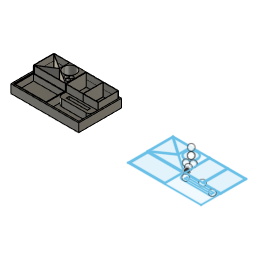
Desk Organizer v13 (Autodesk Fusion 360 design; units mm, degrees)
Autodesk Fusion 360 part; units mm, degrees
sketch "Sketch1" plane through (0, 0, 0) normal (0, 0, 1) x (1, 0, 0)
  line L0 (125, -80) -> (-125, -80)
  line L1 (-125, -80) -> (-125, 80)
  line L2 (-125, 80) -> (125, 80)
  line L3 (125, 80) -> (125, -80)
  line L4 (125, -80) -> (-125, 80) construction
  line L5 (-125, -80) -> (125, 80) construction
  dimension "d1" = 250
  constraint horizontal L0
  constraint perpendicular L0 L1
  constraint parallel L0 L2
  constraint parallel L1 L3
  constraint coincident L4 origin
  constraint coincident L5 origin
  measures "d1" distance of L1.end L2.end
extrude "Extrude1" add sketch "Sketch1" along normal blind 30 makes body 1
sketch "Sketch2" plane through (0, 0, 30) normal (0, 0, 1) x (-1, 0, 0)
  line L0 (-125, -80) -> (125, -80)
  line L1 (125, -80) -> (125, 80)
  line L2 (125, 80) -> (-125, 80)
  line L3 (-125, 80) -> (-125, -80)
  line L4 (119.192, -76.1203) -> (-119.192, -76.1203)
  line L5 (-119.192, -76.1203) -> (-119.192, 76.1203)
  line L6 (-119.192, 76.1203) -> (119.192, 76.1203)
  line L7 (119.192, 76.1203) -> (119.192, -76.1203)
  line L8 (119.192, -76.1203) -> (-119.192, 76.1203) construction
  line L9 (-119.192, -76.1203) -> (119.192, 76.1203) construction
  constraint horizontal L4
  constraint perpendicular L4 L5
  constraint parallel L4 L6
  constraint parallel L5 L7
  constraint coincident L8 origin
  constraint coincident L9 origin
extrude "Extrude2" cut sketch "Sketch2" against normal blind 26 contours L4 L5 L6 L7 bodies 1
sketch "Sketch3" plane through (0, 0, 4) normal (0, 0, 1) x (-1, 0, 0)
  line L0 (119.192, 76.1203) -> (-119.192, 76.1203)
  line L1 (-119.192, 76.1203) -> (-119.192, -76.1203)
  line L2 (-119.192, -76.1203) -> (119.192, -76.1203)
  line L3 (119.192, -76.1203) -> (119.192, 76.1203)
  line L4 (2.1554, -1.5872) -> (116.2965, -1.5872)
  line L5 (116.2965, -1.5872) -> (116.2965, -74.3239)
  line L6 (116.2965, -74.3239) -> (2.1554, -74.3239)
  line L7 (2.1554, -74.3239) -> (2.1554, -1.5872)
  line L8 (2.1554, -1.5872) -> (116.2965, -74.3239) construction
  line L9 (116.2965, -1.5872) -> (2.1554, -74.3239) construction
  point P0 (59.2259, -37.9555)
  constraint horizontal L4
  constraint perpendicular L4 L5
  constraint parallel L4 L6
  constraint parallel L5 L7
  constraint coincident L8 P0
  constraint coincident L9 P0
extrude "Extrude3" add sketch "Sketch3" along normal blind 50 separate body contours L4 L5 L6 L7 makes body 2
sketch "Sketch4" plane through (0, 0, 30) normal (0, 0, 1) x (-1, 0, 0)
  line L0 (-119.192, -76.1203) -> (-119.192, 76.1203)
  line L1 (-119.192, 76.1203) -> (119.192, 76.1203)
  line L2 (119.192, 76.1203) -> (119.192, -76.1203)
  line L3 (119.192, -76.1203) -> (-119.192, -76.1203)
  line L4 (-125, -80) -> (125, -80)
  line L5 (125, -80) -> (125, 80)
  line L6 (125, 80) -> (-125, 80)
  line L7 (-125, 80) -> (-125, -80)
sketch "Sketch5" plane through (0, 0, 54) normal (0, 0, 1) x (-1, 0, 0)
  line L0 (2.1554, -74.3239) -> (116.2965, -74.3239)
  line L1 (116.2965, -74.3239) -> (116.2965, -1.5872)
  line L2 (116.2965, -1.5872) -> (2.1554, -1.5872)
  line L3 (2.1554, -1.5872) -> (2.1554, -74.3239)
  line L4 (115, -72.3079) -> (115, -2.8697)
  line L5 (115, -2.8697) -> (5, -2.8697)
  line L6 (5, -2.8697) -> (5, -72.3079)
  line L7 (5, -72.3079) -> (115, -72.3079)
  line L8 (115, -72.3079) -> (5, -2.8697)
  line L9 (5, -72.3079) -> (115, -2.8697)
  constraint parallel L1 L4
  constraint perpendicular L4 L5
  constraint perpendicular L5 L6
  constraint perpendicular L4 L7
extrude "Extrude4" cut sketch "Sketch5" against normal blind 45 contours L4 L8 L9 bodies 2
sketch "Sketch6" plane through (0, 0, 54) normal (0, 0, 1) x (-1, 0, 0)
  line L0 (60, -37.5888) -> (115, -2.8697)
  line L1 (115, -2.8697) -> (115, -72.3079)
  line L2 (115, -72.3079) -> (60, -37.5888)
  line L3 (2.1554, -74.3239) -> (116.2965, -74.3239)
  line L4 (116.2965, -74.3239) -> (116.2965, -1.5872)
  line L5 (116.2965, -1.5872) -> (2.1554, -1.5872)
  line L6 (2.1554, -1.5872) -> (2.1554, -74.3239)
  line L7 (59.2259, -37.1001) -> (3.961, -2.9832)
  line L8 (3.961, -2.9832) -> (113.0235, -2.8515)
  line L9 (113.0235, -2.8515) -> (59.2259, -37.1001)
extrude "Extrude5" cut sketch "Sketch6" against normal blind 45 contours L7 L8 L9 bodies 2
sketch "Sketch7" plane through (0, 0, 54) normal (0, 0, 1) x (-1, 0, 0)
  line L0 (59.2259, -37.1001) -> (3.961, -2.9832)
  line L1 (3.961, -2.9832) -> (113.0235, -2.8515)
  line L2 (113.0235, -2.8515) -> (59.2259, -37.1001)
  line L3 (60, -37.5888) -> (115, -2.8697)
  line L4 (115, -2.8697) -> (115, -72.3079)
  line L5 (115, -72.3079) -> (60, -37.5888)
  line L6 (2.1554, -74.3239) -> (116.2965, -74.3239)
  line L7 (116.2965, -74.3239) -> (116.2965, -1.5872)
  line L8 (116.2965, -1.5872) -> (2.1554, -1.5872)
  line L9 (2.1554, -1.5872) -> (2.1554, -74.3239)
  line L10 (60, -38.3558) -> (60, -73.2667)
  line L11 (60, -73.2667) -> (115, -73.2667)
  line L12 (115, -73.2667) -> (60, -38.3558)
  constraint vertical L10
  constraint perpendicular L10 L11
extrude "Extrude6" cut sketch "Sketch7" against normal blind 45 contours L10 L11 L12 bodies 2
sketch "Sketch8" plane through (0, 0, 54) normal (0, 0, 1) x (-1, 0, 0)
  line L0 (60, -73.2667) -> (60, -38.3558)
  line L1 (60, -38.3558) -> (115, -73.2667)
  line L2 (115, -73.2667) -> (60, -73.2667)
  line L3 (59.2259, -37.1001) -> (3.961, -2.9832)
  line L4 (3.961, -2.9832) -> (113.0235, -2.8515)
  line L5 (113.0235, -2.8515) -> (59.2259, -37.1001)
  line L6 (60, -37.5888) -> (115, -2.8697)
  line L7 (115, -2.8697) -> (115, -72.3079)
  line L8 (115, -72.3079) -> (60, -37.5888)
  line L9 (2.1554, -74.3239) -> (116.2965, -74.3239)
  line L10 (116.2965, -74.3239) -> (116.2965, -1.5872)
  line L11 (116.2965, -1.5872) -> (2.1554, -1.5872)
  line L12 (2.1554, -1.5872) -> (2.1554, -74.3239)
  circle A0 centre (35.6462, -50.553) radius 22.3607
extrude "Extrude7" cut sketch "Sketch8" against normal blind 45 contours A0 bodies 2
move_body "Move1" bodies 2 to x (1, 0, 0) y (0, 1, 0) z (0, 0, 1) at (283.173, -5.0322, 0)
sketch "Sketch9" plane through (0, 0, 54) normal (0, 0, 1) x (-1, 0, 0)
  circle A0 centre (-247.5268, -45.5208) radius 22.3607
  line L0 (-223.173, -68.2344) -> (-223.173, -33.3236)
  line L1 (-223.173, -33.3236) -> (-168.173, -68.2344)
  line L2 (-168.173, -68.2344) -> (-223.173, -68.2344)
  line L3 (-223.947, -32.0679) -> (-279.212, 2.049)
  line L4 (-279.212, 2.049) -> (-170.1495, 2.1807)
  line L5 (-170.1495, 2.1807) -> (-223.947, -32.0679)
  line L6 (-223.173, -32.5565) -> (-168.173, 2.1626)
  line L7 (-168.173, 2.1626) -> (-168.173, -67.2756)
  line L8 (-168.173, -67.2756) -> (-223.173, -32.5565)
  line L9 (-281.0176, -69.2917) -> (-166.8765, -69.2917)
  line L10 (-166.8765, -69.2917) -> (-166.8765, 3.4451)
  line L11 (-166.8765, 3.4451) -> (-281.0176, 3.4451)
  line L12 (-281.0176, 3.4451) -> (-281.0176, -69.2917)
  circle A1 centre (-261.4315, -18.5457) radius 6.2199
  circle A2 centre (-272.1085, -27.4432) radius 6.2744
  circle A3 centre (-273.71, -12.3175) radius 6.3191
extrude "Extrude8" cut sketch "Sketch9" against normal blind 45 contours A1 | A2 | A3 bodies 2
move_body "Move2" bodies 2 to x (1, 0, 0) y (0, 1, 0) z (0, 0, 1) at (-284.7373, 5.4237, 0)
sketch "Sketch10" plane through (0, 0, 54) normal (0, 0, 1) x (-1, 0, 0)
  circle A0 centre (12.6289, -32.8669) radius 6.2744
  circle A1 centre (23.3058, -23.9694) radius 6.2199
  circle A2 centre (11.0273, -17.7412) radius 6.3191
  circle A3 centre (37.2105, -50.9445) radius 22.3607
  line L0 (61.5643, -73.6581) -> (61.5643, -38.7472)
  line L1 (61.5643, -38.7472) -> (116.5643, -73.6581)
  line L2 (116.5643, -73.6581) -> (61.5643, -73.6581)
  line L3 (60.7903, -37.4916) -> (5.5253, -3.3747)
  line L4 (5.5253, -3.3747) -> (114.5878, -3.2429)
  line L5 (114.5878, -3.2429) -> (60.7903, -37.4916)
  line L6 (61.5643, -37.9802) -> (116.5643, -3.2611)
  line L7 (116.5643, -3.2611) -> (116.5643, -72.6993)
  line L8 (116.5643, -72.6993) -> (61.5643, -37.9802)
  line L9 (3.7197, -74.7154) -> (117.8608, -74.7154)
  line L10 (117.8608, -74.7154) -> (117.8608, -1.9786)
  line L11 (117.8608, -1.9786) -> (3.7197, -1.9786)
  line L12 (3.7197, -1.9786) -> (3.7197, -74.7154)
  line L13 (-116.6264, -1.9786) -> (-1.9597, -1.9786)
  line L14 (-1.9597, -1.9786) -> (-1.9597, -74.7154)
  line L15 (-1.9597, -74.7154) -> (-116.6264, -74.7154)
  line L16 (-116.6264, -74.7154) -> (-116.6264, -1.9786)
  line L17 (-116.6264, -1.9786) -> (-1.9597, -74.7154) construction
  line L18 (-1.9597, -1.9786) -> (-116.6264, -74.7154) construction
  point P0 (-59.2931, -38.347)
  constraint horizontal L13
  constraint perpendicular L13 L14
  constraint parallel L13 L15
  constraint parallel L14 L16
  constraint coincident L17 P0
  constraint coincident L18 P0
  constraint midpoint L17 P0
extrude "Extrude9" add sketch "Sketch10" against normal blind 49 separate body contours L13 L14 L15 L16 makes body 3
sketch "Sketch11" plane through (0, 0, 54) normal (0, 0, 1) x (-1, 0, 0)
  line L0 (-116.6264, -74.7154) -> (-1.9597, -74.7154)
  line L1 (-1.9597, -74.7154) -> (-1.9597, -1.9786)
  line L2 (-1.9597, -1.9786) -> (-116.6264, -1.9786)
  line L3 (-116.6264, -1.9786) -> (-116.6264, -74.7154)
  line L4 (-3.5608, -73.4896) -> (-62.607, -73.4896)
  line L5 (-62.607, -73.4896) -> (-62.607, -3.1642)
  line L6 (-62.607, -3.1642) -> (-3.5608, -3.1642)
  line L7 (-3.5608, -3.1642) -> (-3.5608, -73.4896)
  constraint horizontal L4
  constraint vertical L5
  constraint horizontal L6
  constraint vertical L7
extrude "Extrude10" cut sketch "Sketch11" against normal blind 45 contours L4 L5 L6 L7 bodies 3
sketch "Sketch12" plane through (0, 0, 54) normal (0, 0, 1) x (-1, 0, 0)
  line L0 (-62.607, -73.4896) -> (-62.607, -3.1642)
  line L1 (-62.607, -3.1642) -> (-3.5608, -3.1642)
  line L2 (-3.5608, -3.1642) -> (-3.5608, -73.4896)
  line L3 (-3.5608, -73.4896) -> (-62.607, -73.4896)
  line L4 (-116.6264, -74.7154) -> (-1.9597, -74.7154)
  line L5 (-1.9597, -74.7154) -> (-1.9597, -1.9786)
  line L6 (-1.9597, -1.9786) -> (-116.6264, -1.9786)
  line L7 (-116.6264, -1.9786) -> (-116.6264, -74.7154)
  line L8 (-63.6611, -73.4896) -> (-116, -73.4896)
  line L9 (-116, -73.4896) -> (-116, -3.3521)
  line L10 (-116, -3.3521) -> (-63.6611, -3.3521)
  line L11 (-63.6611, -3.3521) -> (-63.6611, -73.4896)
  constraint horizontal L8
  constraint vertical L9
  constraint horizontal L10
  constraint vertical L11
extrude "Extrude11" cut sketch "Sketch12" against normal blind 45 contours L8 L9 L10 L11 bodies 3
sketch "Sketch13" plane through (0, 0, 30) normal (0, 0, 1) x (-1, 0, 0)
  line L0 (-3.0546, 2.517) -> (-115, 2.517)
  line L1 (-115, 2.517) -> (-115, 17.5)
  line L2 (-102.5, 30) -> (-15.5546, 30)
  line L3 (-3.0546, 17.5) -> (-3.0546, 2.517)
  arc A0 (-3.0546, 17.5) -> (-15.5546, 30) centre (-15.5546, 17.5) ccw
  arc A1 (-102.5, 30) -> (-115, 17.5) centre (-102.5, 17.5) ccw
  dimension "d24" = 12.5
  constraint horizontal L0
  constraint vertical L1
  constraint horizontal L2
  constraint vertical L3
  constraint tangent L2 A0
  constraint tangent L3 A0
  constraint tangent L1 A1
  constraint tangent L2 A1
  constraint equal A0 A1
  measures "d24" radius of A0
extrude "Extrude12" add sketch "Sketch13" against normal blind 25 separate body makes body 4
sketch "Sketch14" plane through (0, 0, 30) normal (0, 0, 1) x (-1, 0, 0)
  line L0 (-22.0307, 10) -> (-97.0307, 10)
  line L1 (-97.0307, 10) -> (-97.0307, 20)
  line L2 (-97.0307, 20) -> (-22.0307, 20)
  line L3 (-22.0307, 20) -> (-22.0307, 10)
  constraint horizontal L0
  constraint vertical L1
  constraint horizontal L2
  constraint vertical L3
extrude "Extrude13" cut sketch "Sketch14" against normal blind 20 bodies 4
sketch "Sketch15" plane through (0, 0, 30) normal (0, 0, 1) x (-1, 0, 0)
  line L0 (116.1282, 2.9693) -> (1.7275, 2.9693)
  line L1 (1.7275, 2.9693) -> (1.7275, 73.433)
  line L2 (1.7275, 73.433) -> (116.1282, 73.433)
  line L3 (116.1282, 73.433) -> (116.1282, 2.9693)
  constraint horizontal L0
  constraint vertical L1
  constraint horizontal L2
  constraint vertical L3
sketch "Sketch16" plane through (0, 0, 30) normal (0, 0, 1) x (-1, 0, 0)
  line L0 (113.46, 5.4) -> (5.0422, 5.4)
  line L1 (5.0422, 5.4) -> (5.0422, 70.1017)
  line L2 (5.0422, 70.1017) -> (113.46, 70.1017)
  line L3 (113.46, 70.1017) -> (113.46, 5.4)
  constraint horizontal L0
  constraint vertical L1
  constraint horizontal L2
  constraint vertical L3
move_body "Move3" bodies 1 to x (1, 0, 0) y (0, 1, 0) z (0, 0, 1) at (-266.4429, 0, 1.5616)
move_body "Move4" bodies 2 to x (1, 0, 0) y (0, 1, 0) z (0, 0, 1) at (-55.2047, 106.1335, 0)
move_body "Move5" bodies 3 to x (1, 0, 0) y (0, 1, 0) z (0, 0, 1) at (-11.6109, 104.6452, 0)
move_body "Move6" bodies 4 to x (1, 0, 0) y (0, 1, 0) z (0, 0, 1) at (5.9394, -97.6743, 0)
move_body "Move8" bodies 3 to x (1, 0, 0) y (0, 1, 0) z (0, 0, 1) at (-255.7495, -105.647, 0)
move_body "Move9" bodies 2 to x (1, 0, 0) y (0, 1, 0) z (0, 0, 1) at (-209.1872, -107.0558, 0)
move_body "Move11" bodies 4 to x (1, 0, 0) y (0, 1, 0) z (0, 0, 1) at (-273.4479, 96.4393, 0)
move_body "Move12" bodies 2 to x (1, 0, 0) y (0, 1, 0) z (0, 0, 1) at (-2.937, 1.7568, 0)
move_body "Move13" bodies 3 to x (1, 0, 0) y (0, 1, 0) z (0, 0, 1) at (-4.7566, 1.6446, 0)
move_body "Move15" bodies 4 to x (1, 0, 0) y (0, 1, 0) z (0, 0, 1) at (-4.1785, 5.2913, 0)
move_face "OffsetFaces1" offset 7 1 faces at (-147.2509, 25.3734, 22.8949) on bodies 1
move_face "OffsetFaces2" offset -8 1 faces at (-141.4429, 26.6667, 11.5616) on bodies 1
move_face "OffsetFaces3" offset -1 1 faces at (-391.4429, -26.6667, 11.5616) on bodies 1
move_face "OffsetFaces4" offset 9 1 faces at (-231.3789, -76.1203, 22.8949) on bodies 1
move_face "OffsetFaces5" offset -8 1 faces at (-229.7762, -80, 21.5616) on bodies 1
sketch "Sketch17" plane through (0, 0, 5.5616) normal (0, 0, 1) x (-1, 0, 0)
  line L0 (385.6348, 67.1203) -> (154.2509, 67.1203)
  line L1 (154.2509, 67.1203) -> (154.2509, -76.1203)
  line L2 (154.2509, -76.1203) -> (385.6348, -76.1203)
  line L3 (385.6348, -76.1203) -> (385.6348, 67.1203)
  line L4 (385, -2) -> (271, -2)
  line L5 (271, -2) -> (271, 66.2697)
  line L6 (271, 66.2697) -> (385, 66.2697)
  line L7 (385, 66.2697) -> (385, -2)
  constraint horizontal L4
  constraint vertical L5
  constraint horizontal L6
  constraint vertical L7
extrude "Extrude16" add sketch "Sketch17" along normal blind 25 separate body contours L4 L5 L6 L7 makes body 5
move_body "Move17" bodies 5 to x (1, 0, 0) y (0, 1, 0) z (0, 0, 1) at (-11.9716, -62.1549, -50.1833)
move_body "Move18" bodies 5 to x (1, 0, 0) y (0, 1, 0) z (0, 0, 1) at (-119.3378, 20.5362, 0)
sketch "Sketch18" plane through (0, 0, -19.6217) normal (0, 0, 1) x (-1, 0, 0)
  line L0 (516.3095, 107.8885) -> (402.3095, 107.8885)
  line L1 (402.3095, 107.8885) -> (402.3095, 39.6188)
  line L2 (402.3095, 39.6188) -> (516.3095, 39.6188)
  line L3 (516.3095, 39.6188) -> (516.3095, 107.8885)
  line L4 (513.6378, 41.8099) -> (405, 41.8099)
  line L5 (405, 41.8099) -> (405, 106.0721)
  line L6 (405, 106.0721) -> (513.6378, 106.0721)
  line L7 (513.6378, 106.0721) -> (513.6378, 41.8099)
  constraint horizontal L4
  constraint vertical L5
  constraint horizontal L6
  constraint vertical L7
extrude "Extrude17" cut sketch "Sketch18" against normal blind 22 contours L4 L5 L6 L7 bodies 5
move_body "Move19" bodies 5 to x (1, 0, 0) y (0, 1, 0) z (0, 0, 1) at (131.831, 41.6514, 50)
sketch "Sketch19" plane through (0, 0, 0) normal (0, 0, 1) x (1, 0, 0)
  line L0 (288.7232, -75.5137) -> (28.7232, -75.5137)
  line L1 (28.7232, -75.5137) -> (28.7232, 84.4863)
  line L2 (28.7232, 84.4863) -> (288.7232, 84.4863)
  line L3 (288.7232, 84.4863) -> (288.7232, -75.5137)
  line L4 (158.7232, 84.4863) -> (288.7232, 84.4863)
  line L5 (288.7232, 84.4863) -> (288.7232, -5.5137)
  line L6 (288.7232, -5.5137) -> (158.7232, -5.5137)
  line L7 (158.7232, -5.5137) -> (158.7232, 84.4863)
  line L8 (28.7232, 84.4863) -> (158.7232, 84.4863)
  line L9 (158.7232, 84.4863) -> (158.7232, -5.5137)
  line L10 (158.7232, -5.5137) -> (28.7232, -5.5137)
  line L11 (28.7232, -5.5137) -> (28.7232, 84.4863)
  line L12 (28.7232, 84.4863) -> (158.7232, -5.5137)
  line L13 (28.7232, -5.5137) -> (93.7232, 39.4863)
  line L14 (93.7232, 39.4863) -> (93.7232, 84.4863)
  circle A0 centre (119.0143, 58.7272) radius 22.3607
  circle A1 centre (132.504, 27.4364) radius 9.2562
  circle A2 centre (148.2489, 37.2769) radius 8.7724
  circle A3 centre (150.0202, 17.9895) radius 8.6173
  line L15 (223.7232, 84.4863) -> (223.7232, -5.5137)
  line L16 (31.661, -7.9668) -> (157.827, -7.9668)
  line L17 (157.827, -7.9668) -> (157.827, -73.0925)
  line L18 (157.827, -73.0925) -> (31.661, -73.0925)
  line L19 (31.661, -73.0925) -> (31.661, -7.9668)
  line L20 (164.4427, -7.9668) -> (283.7232, -7.9668)
  line L21 (283.7232, -7.9668) -> (283.7232, -18.0137)
  line L22 (271.2232, -30.5137) -> (176.9427, -30.5137)
  line L23 (164.4427, -18.0137) -> (164.4427, -7.9668)
  arc A4 (164.4427, -18.0137) -> (176.9427, -30.5137) centre (176.9427, -18.0137) ccw
  arc A5 (271.2232, -30.5137) -> (283.7232, -18.0137) centre (271.2232, -18.0137) ccw
  point P0 (158.7232, 4.4863)
  dimension "d43" = 12.5
  constraint horizontal L0
  constraint perpendicular L0 L1
  constraint parallel L0 L2
  constraint parallel L1 L3
  constraint horizontal L4
  constraint vertical L5
  constraint horizontal L6
  constraint vertical L7
  constraint coincident L3 L5.end
  constraint midpoint L2 L4.start
  constraint horizontal L8
  constraint vertical L9
  constraint horizontal L10
  constraint vertical L11
  constraint midpoint L12 L13.end
  constraint vertical L14
  constraint midpoint L4 L15.start
  constraint perpendicular L2 L15
  constraint horizontal L16
  constraint vertical L17
  constraint horizontal L18
  constraint vertical L19
  constraint horizontal L20
  constraint vertical L21
  constraint horizontal L22
  constraint vertical L23
  constraint tangent L22 A4
  constraint tangent L23 A4
  constraint tangent L21 A5
  constraint tangent L22 A5
  constraint equal A4 A5
  measures "d43" radius of A4
sketch "Sketch20" plane through (0, 0, 0) normal (0, 0, 1) x (1, 0, 0)
  line L0 (178.7232, -15.5137) -> (273.4079, -15.5137)
  line L1 (273.4079, -15.5137) -> (273.4079, -23.2959)
  line L2 (273.4079, -23.2959) -> (178.7232, -23.2959)
  line L3 (178.7232, -23.2959) -> (178.7232, -15.5137)
  constraint horizontal L0
  constraint vertical L1
  constraint horizontal L2
  constraint vertical L3
sketch "Sketch21" plane through (0, 0, 0) normal (0, 0, 1) x (1, 0, 0)
  line L0 (160.5753, 83.012) -> (221.9971, 83.012)
  line L1 (221.9971, 83.012) -> (221.9971, -4.0433)
  line L2 (221.9971, -4.0433) -> (160.5753, -4.0433)
  line L3 (160.5753, -4.0433) -> (160.5753, 83.012)
  line L4 (225.7232, 82.4863) -> (287.311, 82.4863)
  line L5 (287.311, 82.4863) -> (287.311, -4.0433)
  line L6 (287.311, -4.0433) -> (225.7232, -4.0433)
  line L7 (225.7232, -4.0433) -> (225.7232, 82.4863)
  constraint horizontal L0
  constraint vertical L1
  constraint horizontal L2
  constraint vertical L3
  constraint horizontal L4
  constraint vertical L5
  constraint horizontal L6
  constraint vertical L7
sketch "Sketch22" plane through (0, 0, 0) normal (0, 0, 1) x (1, 0, 0)
  line L0 (30.1224, 81.8292) -> (30.1224, -2.9198)
  line L1 (30.1224, -2.9198) -> (90.7597, 39.1654)
  line L2 (90.7597, 39.1654) -> (30.1224, 81.8292)
  line L3 (31.0732, 84) -> (92, 84)
  line L4 (92, 84) -> (92, 41.3512)
  line L5 (92, 41.3512) -> (31.0732, 84)
  line L6 (93.5492, 38.3781) -> (31.645, -4.2444)
  line L7 (31.645, -4.2444) -> (155.4534, -4.2444)
  line L8 (155.4534, -4.2444) -> (93.5492, 38.3781)
  line L9 (32.63, -8.6225) -> (156.3416, -8.6225)
  line L10 (156.3416, -8.6225) -> (156.3416, -71.8318)
  line L11 (156.3416, -71.8318) -> (32.63, -71.8318)
  line L12 (32.63, -71.8318) -> (32.63, -8.6225)
  circle A0 centre (119, 59) radius 21.1301
  circle A1 centre (132.6412, 27.3411) radius 8.6082
  circle A2 centre (148.2733, 37.2188) radius 8.2897
  circle A3 centre (150, 18) radius 8.2264
  constraint vertical L0
  constraint perpendicular L0 L3
  constraint perpendicular L3 L4
  constraint horizontal L7
  constraint horizontal L9
  constraint vertical L10
  constraint horizontal L11
  constraint vertical L12
